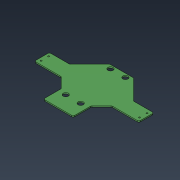
# Autodesk Inventor part: Kickerboard
Saved by Autodesk Inventor 2022.1 (Build 261234020, 234B)
## iProperties
Part Number: Kickerboard
Material: Phenolharz
Document SubType Name: Modeling
Designer: rYan
Mass: 13.1104 g
Surface Area: 126.901 cm^2
Volume: 9.5003 cm^3
Density: 1.38 g/cm^3
Appearance: Glatt - waldgrün
Author: rYan
Autodesk Inventor part; units mm, degrees
ref_plane "YZ Plane" through (0, 0, 0) normal (1, 0, 0) x (0, 1, 0)
ref_plane "XZ Plane" through (0, 0, 0) normal (0, 1, 0) x (-1, 0, 0)
ref_plane "XY Plane" through (0, 0, 0) normal (0, 0, 1) x (1, 0, 0)
sketch "Skizze1" plane through (0, 0, 0) normal (0, 0, 1) x (1, 0, 0)
  line L0 (16, 38) -> (-16, 38)
  line L1 (-20, -23) -> (-20, -47)
  line L2 (-43, 11) -> (-70, 11)
  line L3 (-70, 11) -> (-70, -9)
  line L4 (-70, -9) -> (-34, -9)
  line L5 (43, 11) -> (70, 11)
  line L6 (70, 11) -> (70, -9)
  line L7 (70, -9) -> (34, -9)
  line L8 (-16, 38) -> (-43, 11)
  line L9 (16, 38) -> (43, 11)
  line L10 (20, -23) -> (34, -9)
  line L11 (-34, -9) -> (-20, -23)
  line L12 (20, -47) -> (20, -23)
  line L13 (0, 55) -> (0, -64) projected
  line L14 (-98, 0) -> (98, 0) projected
  line L15 (-70, 1) -> (70, 1) construction
  line L16 (-66, 6) -> (-66, -4) construction
  line L17 (66, 6) -> (66, -4) construction
  circle A0 centre (-66, 6) radius 1
  circle A1 centre (-66, -4) radius 1
  circle A2 centre (66, 6) radius 1
  circle A3 centre (66, -4) radius 1
  line L18 (-10, 33) -> (10, 33) construction
  line L19 (10, 33) -> (10, -27) construction
  line L20 (10, -27) -> (-10, -27) construction
  line L21 (-10, -27) -> (-10, 33) construction
  circle A4 centre (-10, 33) radius 3.5
  circle A5 centre (10, 33) radius 3.5
  circle A6 centre (10, -27) radius 3.5
  circle A7 centre (-10, -27) radius 3.5
  line L22 (-20, -47) -> (20, -47)
  point P0 (0, 0)
  point P1 (-66, 1)
  point P2 (66, 1)
  dimension "d0" = 45
  dimension "d2" = 32
  dimension "d3" = 20
  dimension "d4" = 70
  dimension "d5" = 38
  dimension "d8" = 40
  dimension "d12" = 10
  dimension "d16" = 2
  dimension "d18" = 66
  dimension "d20" = 20
  dimension "d21" = 60
  dimension "d22" = 5
  dimension "d23" = 7
  dimension "d24" = 47
  dimension "d25" = 1
  dimension "d26" = 14
  constraints: 42 end point, 8 centre point, 8 coincident, 6 parallel, 5 perpendicular, 4 horizontal, 4 midpoint, 3 point on line, 2 equal radius, 1 vertical, 12 other
  measures "d0" angle of L8 L2
  measures "d2" distance of L0.start L0.end
  measures "d3" distance of L5.end L6.end
  measures "d4" distance between parallel lines of L13 L6
  measures "d5" distance between parallel lines of L14 L0
  measures "d8" distance between parallel lines of L1 L12
  measures "d12" distance of L16.start L16.end
  measures "d16" diameter of A0
  measures "d18" distance between parallel lines of L13 L16
  measures "d20" distance of L19.end L20.end
  measures "d21" distance of L18.end L19.end
  measures "d22" distance between parallel lines of L0 L18
  measures "d23" diameter of A4
  measures "d24" distance between parallel lines of L22 L14
  measures "d25" distance between parallel lines of L14 L15
  measures "d26" distance from line of L7.end L12
extrude "Extrusion1" add sketch "Skizze1" along normal blind 1.6
fillet "Rundung1" radius 2 14 edges at (-70, -9, 0.8) (-70, 11, 0.8) (70, -9, 0.8) (70, 11, 0.8) (-20, -47, 0.8) (-20, -23, 0.8) (-34, -9, 0.8) (-43, 11, 0.8) (-16, 38, 0.8) (16, 38, 0.8) (43, 11, 0.8) (20, -23, 0.8) (34, -9, 0.8) (20, -47, 0.8)
